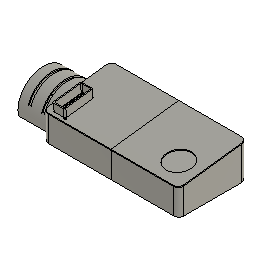
Kontroller v13 (Autodesk Fusion 360 archive; units mm, degrees)
design "Button Panel"
Autodesk Fusion 360 part; units mm, degrees
sketch "Sketch1" plane through (0, 0, 0) normal (1, 0, 0) x (0, 1, 0) in component "Enclosure"
  line L0 (0, 0) -> (200, 0)
  line L1 (200, 0) -> (200, 100)
  line L2 (200, 100) -> (0, 75)
  line L3 (0, 75) -> (0, 0)
  dimension "d1" = 200
  dimension "d2" = 75
  dimension "d37" = 97.125
  constraint vertical L1
  constraint vertical L3
  constraint coincident L0.start L3.end
  measures "d1" distance of L0.start L0.end
  measures "d2" distance of L0.start L2.end
  measures "d37" angle of L2 L3
extrude "Extrude1" add sketch "Sketch1" along normal blind 400 makes body 1 in component "Enclosure"
shell "Shell1" thickness 3 removed faces 1 at (133.3333, 133.3333, 91.6667) on bodies 1 in component "Enclosure"
fillet "Fillet1" radius 15 4 edges at (0, 0, 37.5) (0, 200, 50) (400, 200, 50) (400, 0, 37.5) on bodies 1 in component "Enclosure"
fillet "Fillet1" radius 10 4 edges at (397, 3, 39.1875) (397, 197, 51.3125) (3, 197, 51.3125) (3, 3, 39.1875) on bodies 1 in component "Enclosure"
sketch "Sketch1 (2)" plane through (0, -9.2308, 73.8462) normal (0, -0.124035, 0.992278) x (1, 0, 0) in component "Lid"
  line L0 (387, 12.326) -> (13, 12.326)
  ellipse E0 centre (13, 22.4038) end of major axis (13, 12.326) minor radius 10 (3, 22.4038) -> (13, 12.326) ccw
  line L1 (3, 22.4038) -> (3, 197.7579)
  ellipse E1 centre (13, 197.7579) end of major axis (13, 207.8357) minor radius 10 (13, 207.8357) -> (3, 197.7579) ccw
  line L2 (13, 207.8357) -> (387, 207.8357)
  ellipse E2 centre (387, 197.7579) end of major axis (387, 207.8357) minor radius 10 (397, 197.7579) -> (387, 207.8357) ccw
  line L3 (397, 197.7579) -> (397, 22.4038)
  ellipse E3 centre (387, 22.4038) end of major axis (387, 12.326) minor radius 10 (387, 12.326) -> (397, 22.4038) ccw
  ellipse E4 centre (385, 24.4193) end of major axis (385, 9.3026) minor radius 15 (385, 9.3026) -> (400, 24.4193) ccw
  line L4 (400, 24.4193) -> (400, 195.7423)
  ellipse E5 centre (385, 195.7423) end of major axis (385, 210.859) minor radius 15 (400, 195.7423) -> (385, 210.859) ccw
  line L5 (385, 210.859) -> (15, 210.859)
  ellipse E6 centre (15, 195.7423) end of major axis (15, 210.859) minor radius 15 (15, 210.859) -> (0, 195.7423) ccw
  line L6 (0, 195.7423) -> (0, 24.4193)
  ellipse E7 centre (15, 24.4193) end of major axis (15, 9.3026) minor radius 15 (0, 24.4193) -> (15, 9.3026) ccw
  line L7 (15, 9.3026) -> (385, 9.3026)
extrude "Extrude1'" add sketch "Sketch1 (2)" along normal blind 3 separate body contours L0 E0 L1 E1 L2 E2 L3 E3 | E4 L4 E5 L5 E6 L6 E7 L7 makes body 2 in component "Lid"
sketch "Sketch2" plane through (0, -9.6029, 76.823) normal (0, -0.124035, 0.992278) x (1, 0, 0) in component "Lid"
  circle A0 centre (-60, 100) radius 3
  line L0 (-85, 107.9619) -> (-53.7081, 107.9619) construction
  line L1 (-53.7081, 107.9619) -> (-53.7081, 115) construction
  line L2 (-53.7081, 115) -> (-85, 115) construction
  line L3 (-85, 115) -> (-85, 107.9619) construction
  line L4 (-69.3285, 62.1253) -> (-49.3285, 62.1253)
  line L5 (-49.3285, 62.1253) -> (-49.3285, 50.1253)
  line L6 (-49.3285, 50.1253) -> (-69.3285, 50.1253)
  line L7 (-69.3285, 50.1253) -> (-69.3285, 62.1253)
  line L8 (-90.1362, 68.3274) -> (-65.1362, 68.3274) construction
  line L9 (-65.1362, 68.3274) -> (-65.1362, 82.3274) construction
  line L10 (-65.1362, 82.3274) -> (-90.1362, 82.3274) construction
  line L11 (-90.1362, 82.3274) -> (-90.1362, 68.3274) construction
  circle A1 centre (15, 185) radius 3
  circle A2 centre (35, 185) radius 3
  line L12 (-50, 125) -> (-70, 125)
  line L13 (-70, 125) -> (-70, 127)
  line L14 (-70, 127) -> (-50, 127)
  line L15 (-50, 127) -> (-50, 125)
  line L16 (-68, 135) -> (-68, 127)
  line L17 (-70, 127) -> (-70, 135)
  line L18 (-70, 135) -> (-68, 135)
  line L19 (-68, 133) -> (-50, 133)
  line L20 (-50, 133) -> (-50, 135)
  line L21 (-50, 135) -> (-68, 135)
  line L22 (-83, 138) -> (-63, 138) construction
  line L23 (-63, 138) -> (-63, 146) construction
  line L24 (-63, 146) -> (-83, 146) construction
  line L25 (-83, 146) -> (-83, 138) construction
  line L26 (-68.5, 133.5) -> (-68.5, 126.5)
  line L27 (-68.5, 126.5) -> (-50, 126.5)
  line L28 (-68.5, 133.5) -> (-50, 133.5)
  line L29 (5.5872, 170.4133) -> (23.5872, 170.4133)
  line L30 (5.5872, 178.4133) -> (7.5872, 178.4133)
  line L31 (5.5872, 168.4133) -> (5.5872, 170.4133)
  line L32 (7.5872, 176.4133) -> (23.5872, 176.4133)
  line L33 (5.5872, 170.4133) -> (5.5872, 178.4133)
  line L34 (23.5872, 168.4133) -> (5.5872, 168.4133)
  line L35 (7.0872, 176.9133) -> (23.5872, 176.9133)
  line L36 (23.5872, 176.4133) -> (23.5872, 178.4133)
  line L37 (7.5872, 178.4133) -> (7.5872, 170.4133)
  line L38 (7.0872, 176.9133) -> (7.0872, 169.9133)
  line L39 (23.5872, 178.4133) -> (7.5872, 178.4133)
  line L40 (7.0872, 169.9133) -> (23.5872, 169.9133)
  line L41 (23.5872, 170.4133) -> (23.5872, 168.4133)
  line L42 (23.5872, 176.4133) -> (23.5872, 170.4133)
  line L43 (25, 25) -> (50, 25)
  line L44 (50, 25) -> (50, 100)
  line L45 (50, 100) -> (25, 100)
  line L46 (25, 100) -> (25, 25)
  circle A3 centre (337.5, 72.5) radius 37.5
  line L47 (15, 9.3026) -> (385, 9.3026)
  ellipse E0 centre (385, 24.4193) end of major axis (385, 9.3026) minor radius 15 (385, 9.3026) -> (400, 24.4193) ccw
  line L48 (400, 24.4193) -> (400, 195.7423)
  ellipse E1 centre (385, 195.7423) end of major axis (385, 210.859) minor radius 15 (400, 195.7423) -> (385, 210.859) ccw
  line L49 (385, 210.859) -> (15, 210.859)
  ellipse E2 centre (15, 195.7423) end of major axis (15, 210.859) minor radius 15 (15, 210.859) -> (0, 195.7423) ccw
  line L50 (0, 195.7423) -> (0, 24.4193)
  ellipse E3 centre (15, 24.4193) end of major axis (15, 9.3026) minor radius 15 (0, 24.4193) -> (15, 9.3026) ccw
  dimension "d17" = 6
  dimension "d18" = 3
  dimension "d19" = 20
  dimension "d20" = 12
  dimension "d21" = 3
  dimension "d22" = 6
  dimension "d23" = 6
  dimension "d25" = 20
  dimension "d26" = 2
  dimension "d27" = 3
  dimension "d38" = 75
  constraint horizontal L4
  constraint vertical L5
  constraint horizontal L6
  constraint vertical L7
  constraint horizontal L12
  constraint vertical L13
  constraint horizontal L14
  constraint vertical L15
  constraint coincident L14 L16.end
  constraint perpendicular L14 L16
  constraint perpendicular L14 L17
  constraint perpendicular L16 L18
  constraint coincident L16 L19.start
  constraint perpendicular L16 L19
  constraint perpendicular L19 L20
  constraint perpendicular L16 L21
  constraint perpendicular L14 L26
  constraint perpendicular L16 L27
  constraint coincident L15 L27.end
  constraint perpendicular L26 L28
  constraint horizontal L34
  constraint vertical L31
  constraint horizontal L29
  constraint vertical L41
  constraint coincident L37.end L29
  constraint perpendicular L29 L37
  constraint perpendicular L29 L33
  constraint perpendicular L30 L37
  constraint coincident L32.start L37
  constraint perpendicular L32 L37
  constraint perpendicular L32 L36
  constraint perpendicular L37 L39
  constraint perpendicular L29 L38
  constraint perpendicular L37 L40
  constraint coincident L40.end L41
  constraint perpendicular L35 L38
  constraint horizontal L43
  constraint vertical L44
  constraint horizontal L45
  constraint vertical L46
  measures "d17" diameter of A0
  measures "d19" distance of L4.start L4.end
  measures "d20" distance of L4.start L6.end
  measures "d22" diameter of A1
  measures "d23" diameter of A2
  measures "d25" distance of L12.start L12.end
  measures "d26" distance of L12.start L14.end
  measures "d38" diameter of A3
extrude "Extrude6" cut sketch "Sketch2" against normal blind 10 contours L43 L44 L45 L46 | A3 bodies 2 in component "Lid"
ref_plane "WorkPlane1" through (200, 100, 49.0625) normal (-1, 0, 0) x (0, -1, 0)
split "Split1" by plane through (200, 100, 49.0625) normal (-1, 0, 0) bodies 1 makes body 3 at (76.6667, 66.6667, 0) in component "Enclosure"
split "Split1'" by plane through (200, 100, 49.0625) normal (-1, 0, 0) bodies 2 makes body 4 at (150, 96.6657, 87.0832) in component "Lid"
sketch "Sketch2 (2)" plane through (0, 0, 0) normal (-1, 0, 0) x (0, 1, 0) in component "Enclosure"
  line L0 (15, 76.875) -> (15, 0)
  line L1 (15, 0) -> (185, 0)
  line L2 (185, 0) -> (185, 98.125)
  line L3 (185, 98.125) -> (15, 76.875)
  circle A0 centre (100.0404, -15) radius 75
  circle A1 centre (100.0404, -15) radius 71.5
  line L4 (171.166, -7.6931) -> (28.9147, -7.6931)
  line L5 (135, -50) -> (65, -50)
  line L6 (65, -50) -> (65, -3.4074)
  line L7 (135, -3.4074) -> (135, -50)
  line L8 (185, -98.125) -> (185, 0)
  line L9 (185, 0) -> (15, 0)
  line L10 (15, 0) -> (15, -76.875)
  line L11 (15, -76.875) -> (185, -98.125)
  dimension "d56" = 143
  dimension "d57" = 150
  dimension "d59" = 70
  dimension "d82" = 15
  constraint coincident A1 L4.start
  constraint coincident A1 L4.end
  constraint coincident A0.centre A1.centre
  constraint horizontal L4
  measures "d56" diameter of A1
  measures "d57" diameter of A0
  measures "d59" distance of L5.start L5.end
  measures "d82" distance of L1 A0.centre
extrude "Extrude2" add sketch "Sketch2 (2)" along normal blind 100 separate body contours L1 A0 A1 L9 L11 | L1 A1 L4 L9 | A0 L11 makes body 5 in component "Enclosure"
sketch "Sketch3" plane through (0, 0, 7.6931) normal (0, 0, 1) x (1, 0, 0) in component "Enclosure"
  line L0 (0, 171.166) -> (-100, 171.166)
  line L1 (-100, 171.166) -> (-100, 28.9147)
  line L2 (-26.5, 30) -> (-34, 30)
  line L3 (-34, 30) -> (-34, 170)
  line L4 (-34, 170) -> (-26.5, 170)
  line L5 (-26.5, 170) -> (-26.5, 30)
  line L6 (-66, 170) -> (-73.5, 170)
  line L7 (-73.5, 170) -> (-73.5, 30)
  line L8 (-73.5, 30) -> (-66, 30)
  line L9 (-66, 30) -> (-66, 170)
  line L10 (-34, 100) -> (-66, 100)
  line L11 (0, 28.9147) -> (0, 171.166)
  line L12 (-100, 28.9147) -> (0, 28.9147)
  point P0 (-50, 100)
  dimension "d44" = 7.5
  dimension "d45" = 7.5
  dimension "d46" = 140
  dimension "d47" = 140
  dimension "d48" = 16
  dimension "d50" = -50
  constraint horizontal L2
  constraint vertical L3
  constraint horizontal L4
  constraint vertical L5
  constraint horizontal L6
  constraint vertical L7
  constraint horizontal L8
  constraint vertical L9
  constraint midpoint L3 L10.start
  constraint midpoint L9 L10.end
  constraint perpendicular L9 L10
  constraint midpoint L10 P0
  measures "d44" distance of L3.end L4.end
  measures "d45" distance of L6.start L6.end
  measures "d46" distance of L2.start L4.end
  measures "d47" distance of L6.start L8.end
  measures "d48" distance of L3 P0
  measures "d50" distance of L1 P0
extrude "Extrude3" cut sketch "Sketch3" along normal through all contours L2 L3 L4 L5 | L6 L7 L8 L9 bodies 5 3 in component "Enclosure"
extrude "Extrude4" add sketch "Sketch2 (2)" against normal blind 4 from surface at 100 contours A1 L4 L5 L6 L7 | L4 L5 L6 L7 bodies 5 3 in component "Enclosure"
extrude "Extrude5" cut sketch "Sketch2 (2)" against normal up to surface (3 mm away) contours L4 L5 L6 L7 bodies 3 5 in component "Enclosure"
sketch "Sketch1 (3)" plane through (0, -9.6029, 76.823) normal (0, -0.124035, 0.992278) x (1, 0, 0) in component "Translation Lid"
  line L0 (200, 9.3026) -> (200, 210.859)
  line L1 (200, 210.859) -> (15, 210.859)
  ellipse E0 centre (15, 195.7423) end of major axis (15, 210.859) minor radius 15 (15, 210.859) -> (0, 195.7423) ccw
  line L2 (0, 195.7423) -> (0, 24.4193)
  ellipse E1 centre (15, 24.4193) end of major axis (15, 9.3026) minor radius 15 (0, 24.4193) -> (15, 9.3026) ccw
  line L3 (15, 9.3026) -> (200, 9.3026)
  line L4 (50, 25) -> (25, 25)
  line L5 (25, 25) -> (25, 100)
  line L6 (25, 100) -> (50, 100)
  line L7 (50, 100) -> (50, 25)
  line L8 (19.6479, 104.6721) -> (55, 104.6721)
  line L9 (55, 104.6721) -> (55, 19.794)
  line L10 (55, 19.794) -> (19.6479, 19.794)
  line L11 (19.6479, 19.794) -> (19.6479, 104.6721)
  line L12 (23, 102) -> (52, 102)
  line L13 (52, 102) -> (52, 23)
  line L14 (52, 23) -> (23, 23)
  line L15 (23, 23) -> (23, 102)
  line L16 (55.7446, 14.8644) -> (59.9699, 19.1243)
  line L17 (59.9699, 19.1243) -> (55, 24.0539)
  line L18 (55, 24.0539) -> (50.7747, 19.794)
  line L19 (50.7747, 19.794) -> (55.7446, 14.8644)
  line L20 (18.9033, 109.6016) -> (14.678, 105.3417)
  line L21 (14.678, 105.3417) -> (19.6479, 100.4122)
  line L22 (19.6479, 100.4122) -> (23.8732, 104.6721)
  line L23 (23.8732, 104.6721) -> (18.9033, 109.6016)
  dimension "d107" = 7
  dimension "d108" = 6
  dimension "d109" = 6
  dimension "d110" = 7
  constraint horizontal L8
  constraint vertical L9
  constraint horizontal L10
  constraint vertical L11
  constraint horizontal L12
  constraint vertical L13
  constraint horizontal L14
  constraint vertical L15
  constraint perpendicular L16 L17
  constraint parallel L16 L18
  constraint parallel L17 L19
  constraint perpendicular L20 L21
  constraint parallel L20 L22
  constraint parallel L21 L23
  constraint coincident L10 L18.end
  constraint coincident L9 L17.end
  constraint coincident L8 L22.end
  constraint coincident L11 L21.end
  constraint parallel L18 L22
  measures "d107" distance of L16.end L17.end
  measures "d108" distance of L16.start L16.end
  measures "d109" distance of L20.start L20.end
  measures "d110" distance of L20.start L22.end
extrude "Extrude1''" add sketch "Sketch1 (3)" along normal blind 25 separate body contours L8 L9 L10 L11 L18 L22 makes body 6 in component "Translation Lid"
extrude "Extrude2'" add sketch "Sketch1 (3)" along normal blind 1 contours L8 L11 L20 L21 L23 | L8 L11 L22 | L9 L10 L16 L17 L19 | L9 L10 L18 bodies 6 in component "Translation Lid"
fillet "Fillet1'" radius 2.5 6 edges at (19.6479, 8.4878, 91.6816) (23, 11.6691, 92.0793) (23, 90.059, 101.878) (52, 90.059, 101.878) (55, 92.7105, 102.2094) (52, 11.6691, 92.0793) on bodies 6 in component "Translation Lid"
fillet "Fillet2" radius 1 2 edges at (55.7446, 5.0848, 79.1628) (59.9699, 9.3118, 79.6912) on bodies 6 in component "Translation Lid"
fillet "Fillet2" radius 1 2 edges at (14.678, 94.8634, 90.3852) (18.9033, 99.0904, 90.9135) on bodies 6 in component "Translation Lid"
hole "Hole1" at (19.3233, 94.4218, 90.8338) direction (0, 0.124035, -0.992278) diameter 5 depth 10 tip angle 180 bodies 4 in component "Lid"
hole "Hole1'" at (19.3233, 94.4218, 90.8338) direction (0, 0.124035, -0.992278) diameter 5 depth 10 tip angle 180 bodies 6 in component "Translation Lid"
hole "Hole2" at (55.3246, 9.6293, 80.2348) direction (0, 0.124035, -0.992278) diameter 5 depth 10 tip angle 180 bodies 4 in component "Lid"
hole "Hole2'" at (55.3246, 9.6293, 80.2348) direction (0, 0.124035, -0.992278) diameter 5 depth 10 tip angle 180 bodies 6 in component "Translation Lid"
sketch "Sketch4" plane through (0, 0, 7.6931) normal (0, 0, 1) x (1, 0, 0) in component "Enclosure"
  line L0 (0, 135) -> (0, 65)
  line L1 (0, 65) -> (3, 65)
  line L2 (3, 65) -> (3, 135)
  line L3 (3, 135) -> (0, 135)
  line L4 (-66, 171.2645) -> (-66, 105.2645)
  line L5 (-66, 105.2645) -> (-96, 105.2645)
  line L6 (-70.071, 105.109) -> (-66, 105.109)
  line L7 (-66, 105.109) -> (-66, 95.109)
  line L8 (-66, 95.109) -> (-70.071, 95.109)
  line L9 (-70.071, 95.109) -> (-70.071, 105.109)
  dimension "d83" = 66
  dimension "d84" = 30
  dimension "d85" = 10
  constraint horizontal L6
  constraint vertical L7
  constraint horizontal L8
  constraint vertical L9
  measures "d83" distance of L4.start L4.end
  measures "d84" distance of L4.end L5.end
  measures "d85" distance of L6.start L8.end
extrude "Extrude6'" add sketch "Sketch4" along normal blind 15 contours L6 L7 L8 L9 bodies 5 in component "Enclosure"
fillet "Fillet2'" radius 5 2 edges at (-68.0355, 95.109, 22.6931) (-68.0355, 105.109, 22.6931) on bodies 5 in component "Enclosure"
extrude "Extrude7" add 1 faces at (-70.071, 98.4423, 14.3605) along direction (-1, 0, 0) blind 25.95 on bodies 5 bodies 5 in component "Enclosure"
sketch "Sketch1 (4)" plane through (-66, 0, 0) normal (1, 0, 0) x (0, 1, 0)
  arc A0 (105.109, 17.6931) -> (95.109, 17.6931) centre (100.109, 17.6931) ccw
  line L0 (95.109, 17.6931) -> (95.109, 7.6931)
  line L1 (95.109, 7.6931) -> (105.109, 7.6931)
  line L2 (105.109, 7.6931) -> (105.109, 17.6931)
  circle A1 centre (100.109, 17.6931) radius 4.5
  dimension "d100" = 9
  constraint concentric A0 A1
  measures "d100" diameter of A1
extrude "Extrude8" add sketch "Sketch1 (4)" along normal blind 5 contours A1 bodies 5 in component "Enclosure"
sketch "Sketch6" plane through (0, 0, 0) normal (1, 0, 0) x (0, 1, 0) in component "Enclosure"
  line L0 (171.166, 7.6931) -> (28.9147, 7.6931)
  arc A0 (171.166, 7.6931) -> (28.9147, 7.6931) centre (100.0404, 15) ccw
  arc A1 (173.5251, 0) -> (26.5557, 0) centre (100.0404, 15) ccw
  line L1 (26.5557, 0) -> (173.5251, 0)
  circle A2 centre (45, 5) radius 2
  circle A3 centre (155, 5) radius 2
  dimension "d103" = 4
  dimension "d104" = 4
  measures "d103" diameter of A2
  measures "d104" diameter of A3
extrude "Extrude9" add sketch "Sketch6" along normal blind 5 contours A2 | A3 bodies 5 in component "Enclosure"
component "Enclosure" placed x (1, 0, 0) y (0, 1, 0) z (0, 0, 1) at (0, 0, 0)
component "Lid" placed x (1, 0, 0) y (0, 1, 0) z (0, 0, 1) at (0, 0, 0)
component "Translation Lid" placed x (1, 0, 0) y (0, 1, 0) z (0, 0, 1) at (0, 0, 0) in component "Lid"
